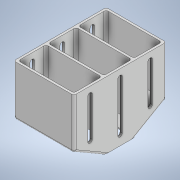
# Autodesk Inventor part: magazine-tower
Saved by Autodesk Inventor 2021 (Build 250183000, 183)
## iProperties
Created: 2024-03-15
Part Number: magazine-tower
Material: Generic
Document SubType Name: Modeling
Designer: 22hamfri
Density: 1 g/cm^3
Appearance: Default
Author: 22hamfri
Autodesk Inventor part; units mm, degrees
ref_plane "YZ Plane" through (0, 0, 0) normal (1, 0, 0) x (0, 1, 0)
ref_plane "XZ Plane" through (0, 0, 0) normal (0, 1, 0) x (-1, 0, 0)
ref_plane "XY Plane" through (0, 0, 0) normal (0, 0, 1) x (1, 0, 0)
sketch "Sketch1" plane through (0, 0, 0) normal (0, 1, 0) x (-1, 0, 0)
  line L0 (-25, 12.5) -> (25, 12.5)
  line L1 (25, 12.5) -> (25, -12.5)
  line L2 (25, -12.5) -> (-25, -12.5)
  line L3 (-25, -12.5) -> (-25, 12.5)
  line L4 (-25, 12.5) -> (25, -12.5) construction
  line L5 (25, 12.5) -> (-25, -12.5) construction
  line L6 (-27, 14.5) -> (27, 14.5)
  line L7 (27, 14.5) -> (27, -14.5)
  line L8 (27, -14.5) -> (-27, -14.5)
  line L9 (-27, -14.5) -> (-27, 14.5)
  line L10 (-27, 14.5) -> (27, -14.5) construction
  line L11 (27, 14.5) -> (-27, -14.5) construction
  point P0 (0, 0)
  dimension "d0" = 25
  dimension "d1" = 50
  dimension "d2" = 2
  dimension "d3" = 2
  constraints: 24 end point, 4 midpoint, 4 parallel, 2 horizontal, 2 perpendicular
  measures "d0" distance between parallel lines of L2 L0
  measures "d1" distance between parallel lines of L3 L1
  measures "d2" distance between parallel lines of L1 L7
  measures "d3" distance between parallel lines of L8 L2
extrude "Extrusion1" add sketch "Sketch1" along normal blind 60
sketch "Sketch2" plane through (27, 0, 14.5) normal (1, 0, 0) x (0, 0, -1)
  line L0 (0, 0) -> (29, 0) projected
  line L1 (29, 0) -> (29, 60) projected
  line L2 (0, 60) -> (29, 60) projected
  line L3 (0, 0) -> (0, 60) projected
  line L4 (27, 0) -> (2, 0) projected
  line L5 (2, 0) -> (2, 60) projected
  line L6 (27, 60) -> (2, 60) projected
  line L7 (27, 0) -> (27, 60) projected
  line L8 (2, 0) -> (2, 60) projected
  line L9 (2, 1.1547) -> (27, 1.1547)
  line L10 (27, 0) -> (27, 60) projected
  line L11 (2, 1.1547) -> (0, 1.1547)
  line L12 (0, 0) -> (0, 60) projected
  line L13 (27, 1.1547) -> (29, 1.1547)
  line L14 (29, 0) -> (29, 60) projected
  line L15 (29, 16.7432) -> (54, 16.7432)
  line L16 (54, 16.7432) -> (56, 16.7432)
  line L17 (54, 16.7432) -> (27, 1.1547)
  line L18 (54, 16.7432) -> (54, 60)
  line L19 (54, 60) -> (29, 60)
  line L20 (54, 60) -> (56, 60)
  line L21 (56, 60) -> (56, 16.7432)
  line L22 (56, 16.7432) -> (56, 15.5885)
  line L23 (56, 15.5885) -> (29, 0)
  line L24 (29, 0) -> (0, 0)
  point P0 (14.5, 0)
  point P1 (29, 2.3094)
  point P2 (29, 0)
  dimension "d6" = 2
  dimension "d8" = 30
  dimension "d15" = 0
  constraints: 26 end point, 8 point on line, 7 perpendicular, 3 parallel, 2 vertical, 1 horizontal
  measures "d6" distance between parallel lines of L23 L17
  measures "d8" angle of L9 L17
  measures "d15" distance between parallel lines of L24 L4
extrude "Extrusion2" add sketch "Sketch2" against normal up to surface (54 mm away) contours L1 L17 L16 L22 L23 | L16 L18 L20 L21
extrude "Extrusion3" add sketch "Sketch2" against normal up to surface (2 mm away) contours L1 L15 L17 | L19 L18 L15 L1
sketch "Sketch3" plane through (-27, 0, -14.5) normal (-1, 0, 0) x (0, 0, 1)
  line L0 (0, 0) -> (29, 0) projected
  line L1 (29, 0) -> (29, 60) projected
  line L2 (0, 60) -> (29, 60) projected
  line L3 (0, 2.3094) -> (0, 60) projected
  line L4 (-25, 16.7432) -> (0, 2.3094) projected
  line L5 (-25, 60) -> (-25, 16.7432) projected
  line L6 (-27, 60) -> (-25, 60) projected
  line L7 (-27, 15.5885) -> (-27, 60) projected
  line L8 (0, 0) -> (-27, 15.5885) projected
  line L9 (0, 60) -> (29, 60) projected
  line L10 (-27, 60) -> (-25, 60) projected
  line L11 (0, 60) -> (-25, 60)
  point P0 (14.5, 0)
  constraints: 2 end point, 1 horizontal
extrude "Extrusion4" add sketch "Sketch3" against normal up to surface (2 mm away) contours L3 L4 L5 L11
sketch "Sketch4" plane through (25, 2.3094, -14.5) normal (-1, 0, 0) x (0, 0, 1)
  line L0 (-25, 57.6906) -> (0, 57.6906) projected
  line L1 (-25, 14.4338) -> (-25, 57.6906) projected
  line L2 (0, 0) -> (-25, 14.4338) projected
  line L3 (0, 57.6906) -> (0, 0) projected
  line L4 (2, -2.3094) -> (27, -2.3094) projected
  line L5 (27, -2.3094) -> (27, 57.6906) projected
  line L6 (2, 57.6906) -> (27, 57.6906) projected
  line L7 (2, -2.3094) -> (2, 57.6906) projected
  line L8 (0, 0) -> (2, -1.1547)
  line L9 (2, -2.3094) -> (2, 57.6906) projected
  line L10 (0, 57.6906) -> (0, 0) projected
  line L11 (0, 11) -> (2, 9.8453)
  point P0 (14.5, -2.3094)
  dimension "d20" = 11
  constraints: 4 end point, 3 point on line, 1 collinear, 1 parallel
  measures "d20" distance of L11.start L2.start
extrude "Extrusion5" cut sketch "Sketch4" along normal up to surface (50 mm away) contours L11 L7 L8 L3
mirror "Mirror1" about plane through (0, 0, 0) normal (0, 0, 1) of "Extrusion2", "Extrusion3", "Extrusion4", "Extrusion5"
fillet "Fillet1" radius 2 12 edges at (25, 36.6547, -14.5) (25, 38.3716, -39.5) (-25, 38.3716, -39.5) (-25, 36.6547, -14.5) (-25, 36.0774, 12.5) (-25, 36.0774, -12.5) (25, 36.0774, -12.5) (25, 36.0774, 12.5) (25, 38.3716, 39.5) (25, 36.6547, 14.5) (-25, 36.6547, 14.5) (-25, 38.3716, 39.5)
fillet "Fillet2" radius 2 4 edges at (-27, 37.7942, -41.5) (27, 37.7942, -41.5) (27, 37.7942, 41.5) (-27, 37.7942, 41.5)
fillet "Fillet3" radius 2 10 edges at (-26.4142, 15.2503, -40.9142) (0, 15.5885, -41.5) (26.4142, 15.2503, -40.9142) (27, 7.2169, -27) (-27, 7.2169, -27) (-26.4142, 15.2503, 40.9142) (0, 15.5885, 41.5) (26.4142, 15.2503, 40.9142) (27, 7.2169, 27) (-27, 7.2169, 27)
sketch "Sketch5" plane through (27, 60, 39.5) normal (1, 0, 0) x (0, 0, -1)
  line L0 (0, 0) -> (0, -43.2568) projected
  line L1 (0, -43.2568) -> (0, 0) projected
  line L2 (25, -46.6906) -> (25, 0) projected
  line L3 (25, 0) -> (25, -46.6906) projected
  line L4 (52, 0) -> (52, -47.8453) projected
  line L5 (52, -47.8453) -> (52, 0) projected
  line L6 (79, -43.2568) -> (79, 0) projected
  line L7 (79, 0) -> (79, -43.2568) projected
  line L8 (27, -47.8453) -> (27, 0) projected
  line L9 (27, 0) -> (27, -47.8453) projected
  line L10 (54, 0) -> (54, -46.6906) projected
  line L11 (54, -46.6906) -> (54, 0) projected
  line L12 (0, -43.2568) -> (0, 0) projected
  line L13 (0, -5) -> (79, -5)
  line L14 (79, 0) -> (79, -43.2568) projected
  line L15 (2, -44.4115) -> (0, -43.2568) projected
  line L16 (0, -43.2568) -> (2, -44.4115) projected
  line L17 (2, -44.4115) -> (27, -58.8453) projected
  line L18 (2, -44.4115) -> (27, -58.8453) projected
  line L19 (79, -43.2568) -> (77, -44.4115) projected
  line L20 (77, -44.4115) -> (52, -58.8453) projected
  line L21 (52, -58.8453) -> (77, -44.4115) projected
  line L22 (77, -44.4115) -> (79, -43.2568) projected
  line L23 (25, -46.6906) -> (25, -57.6906)
  line L24 (29, -60) -> (0, -43.2568) projected
  line L25 (27, -47.8453) -> (27, -58.8453)
  line L26 (52, -47.8453) -> (52, -58.8453)
  line L27 (54, -46.6906) -> (54, -57.6906)
  line L28 (79, -43.2568) -> (50, -60) projected
  line L29 (0, 0) -> (79, 0) projected
  line L30 (29, -60) -> (0, -43.2568) projected
  line L31 (29, -60) -> (50, -60) projected
  line L32 (79, -43.2568) -> (50, -60) projected
  line L33 (79, 0) -> (79, -43.2568) projected
  line L34 (0, 0) -> (79, 0) projected
  line L35 (0, -43.2568) -> (0, 0) projected
  line L36 (27, -53.0718) -> (52, -53.0718)
  line L37 (52, -53.0718) -> (79, -37.4833)
  line L38 (79, -43.2568) -> (79, 0) projected
  line L39 (27, -53.0718) -> (0, -37.4833)
  line L40 (39.5, -53.0718) -> (39.5, -5)
  line L41 (66.5, -5) -> (66.5, -44.7002)
  line L42 (54, -46.6906) -> (54, 0) projected
  line L43 (54, -5) -> (66.5, -5)
  line L44 (66.5, -5) -> (79, -5)
  line L45 (68.5, -5) -> (68.5, -43.5455)
  line L46 (64.5, -5) -> (64.5, -45.8549)
  line L47 (64.5, -5) -> (66.5, -5)
  line L48 (66.5, -5) -> (68.5, -5)
  line L49 (37.5, -5) -> (37.5, -53.0718)
  line L50 (41.5, -53.0718) -> (41.5, -5)
  line L51 (37.5, -5) -> (39.5, -5)
  line L52 (39.5, -5) -> (41.5, -5)
  line L53 (12.5, -5) -> (12.5, -44.7002)
  line L54 (10.5, -5) -> (10.5, -43.5455)
  line L55 (14.5, -5) -> (14.5, -45.8549)
  line L56 (14.5, -5) -> (12.5, -5)
  line L57 (12.5, -5) -> (10.5, -5)
  point P0 (39.5, -60)
  point P1 (10.5, -5)
  point P2 (10.5, -43.5455)
  point P3 (14.5, -5)
  dimension "d26" = 5
  dimension "d27" = 5
  dimension "d28" = 4
  dimension "d29" = 4
  constraints: 50 end point, 31 point on line, 10 symmetric about line, 7 perpendicular, 7 vertical, 6 collinear, 2 midpoint, 10 other
  measures "d26" distance of the line from the sketch origin of L13
  measures "d27" distance between parallel lines of L37 L32
  measures "d28" distance between parallel lines of L50 L49
  measures "d29" distance between parallel lines of L45 L46
extrude "Extrusion6" cut sketch "Sketch5" against normal up to surface (2 mm away) contours L13 L53 L39 L54 | L13 L55 L39 L53 | L13 L40 L36 L49 | L13 L50 L36 L40 | L13 L41 L37 L46 | L13 L45 L37 L41
fillet "Fillet4" radius 2 12 edges at (26, 16.4545, 29) (26, 14.1451, 25) (26, 55, 29) (26, 55, 25) (26, 55, -2) (26, 55, -29) (26, 55, -25) (26, 55, 2) (26, 16.4545, -29) (26, 14.1451, -25) (26, 6.9282, 2) (26, 6.9282, -2)
mirror "Mirror2" about plane through (0, 0, 0) normal (1, 0, 0) of "Extrusion6", "Fillet4"
equation "\"d29\" = d28"
body "Solid1"
